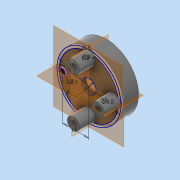
# Autodesk Inventor part: B1cover
Saved by Autodesk Inventor 2022 (Build 260153000, 153)
## iProperties
Created: 2024-04-23
Part Number: B1cover
Material: 一般
Document SubType Name: Modeling
Designer: ktamu
Density: 1 g/cm^3
Appearance: 既定
Author: ktamu
Autodesk Inventor part; units mm, degrees
sketch "BASEscetch" plane through (0, 0, 0) normal (0, 0, 1) x (1, 0, 0)
  circle A0 centre (0, 0) radius 13.5
  circle A1 centre (0, 0) radius 12.4
  circle A2 centre (-11, 0) radius 1.05
  circle A3 centre (0, 0) radius 3
  circle A4 centre (0, 10.4) radius 1.05
  circle A5 centre (0, 10.4) radius 2.6
  circle A6 centre (0, 10.4) radius 2.45
  circle A7 centre (-11, 0) radius 1.8
  point P0 (-12.3418, -1.1998)
  point P1 (-12.3418, 1.1998)
  dimension "d0" = 27
  dimension "d1" = 24.8
  dimension "d2" = 2.1
  dimension "d3" = 11
  dimension "d4" = 6
  dimension "d11" = 2.1
  dimension "d12" = 5.2
  dimension "d13" = 4.9
  dimension "d14" = 0.5
  dimension "d29" = 3.6
  constraints: 8 centre point, 6 coincident
  measures "d0" diameter of A0
  measures "d1" diameter of A1
  measures "d2" diameter of A2
  measures "d3" distance of point (0, 0) A2.centre
  measures "d4" diameter of A3
  measures "d11" diameter of A4
  measures "d12" diameter of A5
  measures "d13" diameter of A6
  measures "d29" diameter of A7
extrude "押し出し1" add sketch "BASEscetch" against normal blind 7.5 contours A0 | A1 A6 A5 | A7 A1 | A1 A6 picked at (-0.2788, 12.8738) picked at (-12.529, 0) picked at (0, 12.5429)
extrude "押し出し3" add sketch "BASEscetch" against normal blind 2 contours A1 A7 A5 | A5 A1 A6 | A1 A7 | A6 A1 | A4 picked at (-2.484, 10.5508) picked at (-12.2217, -0.6961) picked at (0.8846, 11.9857)
extrude "押し出し4" add sketch "BASEscetch" along normal blind 6.5 contours A5 A1 A6 | A1 A6 A5
extrude "押し出し5" add sketch "BASEscetch" along normal blind 6 contours A6 A1 | A1 A6
draft "面の勾配1" angle 1.9 pull direction (0, 0, 1) faces at (2.5663, 9.9829, 4.3333) fixed edges at (-2.6, 10.4, 6.5)
sketch "topScetch" plane through (0, 10.4, 6) normal (0, 0, 1) x (1, 0, 0)
  circle A0 centre (0, 0) radius 1.25
  circle A1 centre (0, 0) radius 2.45
  point P0 (0, -10.4)
  dimension "d20" = 2.5
  constraints: 2 centre point, 1 coincident
  measures "d20" diameter of A0
extrude "押し出し6" add sketch "topScetch" along normal blind 0.5
pattern_circular "円形状パターン1" count 3 over 180 about axis through (0, 0, 0) along (0, 0, -1) of "押し出し4", "押し出し6", "押し出し5", "面の勾配1"
chamfer "面取り1" distance 1 angle 45 1 edges at (-13.5, 0, 0)
extrude "押し出し7" add sketch "BASEscetch" along normal blind 0.04 contours A7 A1 | A1 A7
extrude "押し出し8" add sketch "BASEscetch" against normal blind 0.46 contours A7 A1 picked at (-12.529, 0)
